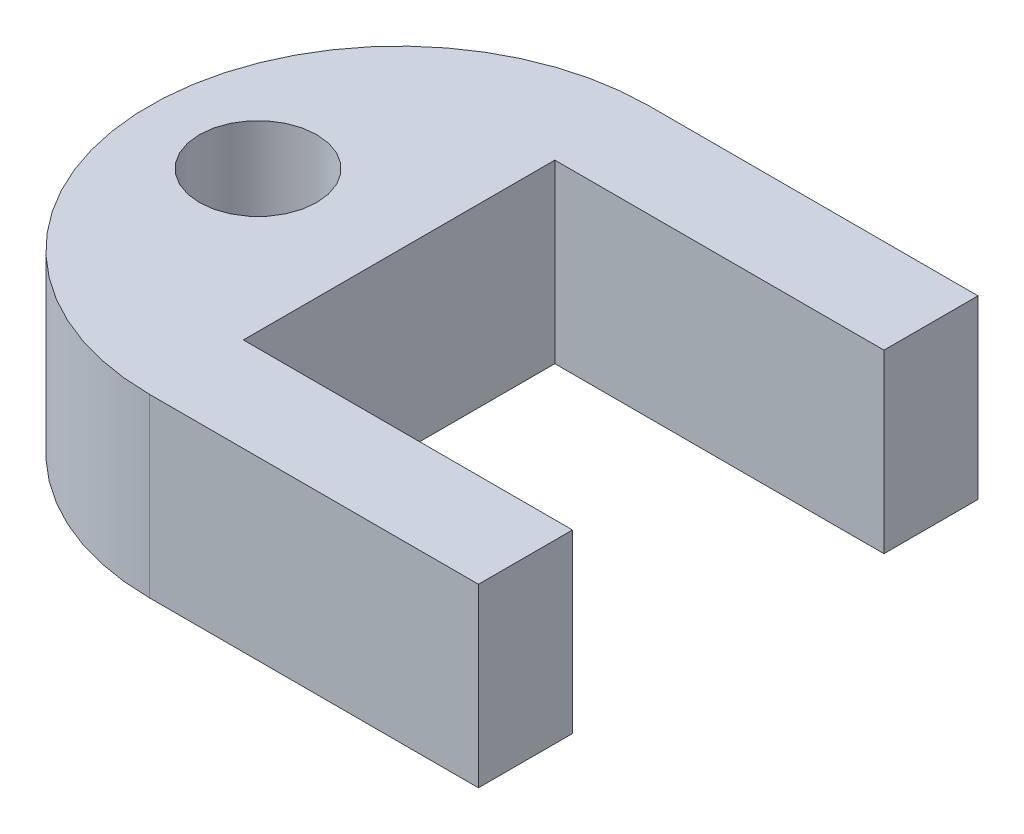
# Autodesk Inventor part: giunto_barra_estrusore
Saved by Autodesk Inventor 2014 SP1 (Build 180222100, 222)
## iProperties
Created: 2015-04-15
Part Number: giunto_barra_estrusore
Material: Generic
Document SubType Name: Modeling
Designer: Giorgio Nuzzo
Density: 1 g/cm^3
Appearance: Default
Author: Giorgio Nuzzo
Autodesk Inventor part; units mm, degrees
ref_plane "YZ Plane" through (0, 0, 0) normal (1, 0, 0) x (0, 1, 0)
ref_plane "XZ Plane" through (0, 0, 0) normal (0, 1, 0) x (-1, 0, 0)
ref_plane "XY Plane" through (0, 0, 0) normal (0, 0, 1) x (1, 0, 0)
sketch "Sketch1" plane through (0, 0, 0) normal (0, 1, 0) x (-1, 0, 0)
  circle A0 centre (0, 0) radius 5
  line L0 (-12, 13.25) -> (-12, -13.25)
  line L1 (-49.85, 0) -> (19.1, 0) construction
  arc A1 (-12, -21.25) -> (-12, 21.25) centre (-12, 0) ccw
  line L2 (-12, -21.25) -> (-40, -21.25)
  line L3 (-40, -21.25) -> (-40, -13.25)
  line L4 (-40, -13.25) -> (-12, -13.25)
  line L5 (-12, 21.25) -> (-40, 21.25)
  line L6 (-40, 21.25) -> (-40, 13.25)
  line L7 (-40, 13.25) -> (-12, 13.25)
  dimension "d0" = 10
  dimension "d1" = 42.5
  dimension "d2" = 12
  dimension "d3" = 8
  dimension "d4" = 28
  dimension "d5" = 21.25
  constraints: 14 end point, 4 symmetric about line, 2 centre point, 2 point on circle, 1 coincident, 1 horizontal, 1 midpoint, 1 parallel, 1 perpendicular, 1 point on line, 1 vertical
  measures "d0" diameter of A0
  measures "d1" distance of L5.start L2.start
  measures "d2" distance from line of point (0, 0) L0
  measures "d3" distance between parallel lines of L2 L4
  measures "d4" distance between parallel lines of L0 L3
  measures "d5" radius of A1
extrude "Extrusion1" add sketch "Sketch1" along normal blind 15
body "Solid1"
